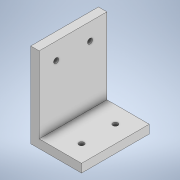
# Autodesk Inventor part: moter support
Saved by Autodesk Inventor 2021 (Build 250183000, 183)
## iProperties
Created: 2024-02-09
Part Number: moter support
Material: Generic
Document SubType Name: Modeling
Designer: haris
Density: 1 g/cm^3
Appearance: Default
Author: haris
Autodesk Inventor part; units mm, degrees
ref_plane "YZ Plane" through (0, 0, 0) normal (1, 0, 0) x (0, 1, 0)
ref_plane "XZ Plane" through (0, 0, 0) normal (0, 1, 0) x (-1, 0, 0)
ref_plane "XY Plane" through (0, 0, 0) normal (0, 0, 1) x (1, 0, 0)
sketch "Sketch1" plane through (0, 0, 0) normal (0, 0, 1) x (1, 0, 0)
  line L0 (0, 0) -> (0, 50)
  line L1 (0, 50) -> (5, 50)
  line L2 (5, 50) -> (5, 5)
  line L3 (5, 5) -> (30, 5)
  line L4 (30, 5) -> (30, 0)
  line L5 (30, 0) -> (0, 0)
  dimension "d0" = 50
  dimension "d1" = 5
  dimension "d2" = 45
  dimension "d3" = 25
  dimension "d4" = 5
  constraints: 12 end point, 3 perpendicular, 1 parallel, 1 vertical
  measures "d0" distance of L0.start L0.end
  measures "d1" distance of L0.end L1.end
  measures "d2" distance of L1.end L2.end
  measures "d3" distance of L2.end L3.end
  measures "d4" distance of L3.end L4.end
extrude "Extrusion1" add sketch "Sketch1" along normal blind 40
sketch "Sketch2" plane through (0, 0, 0) normal (-1, 0, 0) x (0, 0, 1)
  circle A0 centre (10, 40) radius 1.5
  circle A1 centre (30, 40) radius 1.5
  point P0 (0, 0)
  dimension "d7" = 3
  dimension "d8" = 3
  constraints: 2 centre point
  measures "d7" diameter of A0
  measures "d8" diameter of A1
sketch "Sketch3" plane through (0, 0, 0) normal (-1, 0, 0) x (0, 0, 1)
  point P0 (0, 0)
extrude "Extrusion2" cut sketch "Sketch2" against normal through all
sketch "Sketch4" plane through (5, 5, 0) normal (0, 1, 0) x (1, 0, 0)
  point P0 (-5, 0)
sketch "Sketch5" plane through (0, 0, 0) normal (0, -1, 0) x (1, 0, 0)
  circle A0 centre (20, 30) radius 1.5
  circle A1 centre (20, 10) radius 1.5
  point P0 (0, 0)
  dimension "d11" = 3
  dimension "d12" = 3
  constraints: 2 centre point
  measures "d11" diameter of A0
  measures "d12" diameter of A1
extrude "Extrusion3" cut sketch "Sketch5" against normal through all
body "Solid1"
